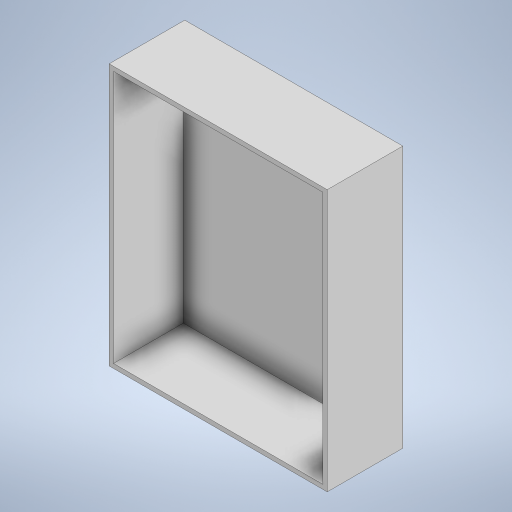
# Autodesk Inventor part: obudowa
Saved by Autodesk Inventor 2023 (Build 270158000, 158)
## iProperties
Created: 2022-11-15
Part Number: obudowa
Material: Generic
Document SubType Name: Modeling
Designer: Kamil
Density: 1 g/cm^3
Appearance: Default
Author: Kamil
Autodesk Inventor part; units mm, degrees
ref_plane "YZ Plane" through (0, 0, 0) normal (1, 0, 0) x (0, 1, 0)
ref_plane "XZ Plane" through (0, 0, 0) normal (0, 1, 0) x (-1, 0, 0)
ref_plane "XY Plane" through (0, 0, 0) normal (0, 0, 1) x (1, 0, 0)
sketch "Sketch5" plane through (0, 0, 0) normal (0, 0, 1) x (1, 0, 0)
  line L0 (0, 0) -> (150, 0)
  line L1 (150, 0) -> (150, 180)
  line L2 (150, 180) -> (0, 180)
  line L3 (0, 180) -> (0, 0)
  line L4 (3, 177) -> (147, 177)
  line L5 (147, 177) -> (147, 3)
  line L6 (147, 3) -> (3, 3)
  line L7 (3, 3) -> (3, 177)
  dimension "d43" = 150
  dimension "d44" = 180
  dimension "d45" = 3
  constraints: 16 end point, 4 parallel, 2 perpendicular, 1 horizontal, 3 other
  measures "d43" distance of L2.end L1.end
  measures "d44" distance of L1.end L0.end
  measures "d45" distance between parallel lines of L2 L4
extrude "Extrusion6" add sketch "Sketch5" against normal blind 4 contours L3 L2 L1 L0 | L4 L5 L6 L7
extrude "Extrusion7" add sketch "Sketch5" along normal blind 48
body "Solid2"
